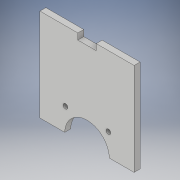
# Autodesk Inventor part: side_plate_top
Saved by Autodesk Inventor 2017 (Build 210142000, 142)
## iProperties
Created: 2017-07-18
Part Number: side_plate_top
Material: Generic
Document SubType Name: Modeling
Designer: millerid
Density: 1 g/cm^3
Appearance: Default
Author: millerid
Autodesk Inventor part; units mm, degrees
ref_plane "YZ Plane" through (0, 0, 0) normal (1, 0, 0) x (0, 1, 0)
ref_plane "XZ Plane" through (0, 0, 0) normal (0, 1, 0) x (-1, 0, 0)
ref_plane "XY Plane" through (0, 0, 0) normal (0, 0, 1) x (1, 0, 0)
sketch "Sketch1" plane through (0, 0, 0) normal (0, 0, 1) x (1, 0, 0)
  line L0 (20.2032, 59.7234) -> (20.2032, 63)
  line L1 (20.2032, 63) -> (0, 63)
  line L2 (0, 63) -> (0, 60)
  line L3 (30, 59.7234) -> (30, 63)
  line L4 (30, 63) -> (50.2032, 63)
  line L5 (50.2032, 63) -> (50.2032, 60)
  line L6 (30, 59.7234) -> (20.2032, 59.7234)
  circle A0 centre (13.6016, 25.8766) radius 1.25
  circle A1 centre (36.5, 25.6) radius 1.25
  line L7 (20.2032, 59.7234) -> (20.2032, 63)
  line L8 (20.2032, 63) -> (0, 63)
  line L9 (0, 63) -> (0, 60)
  line L10 (30, 59.7234) -> (30, 63)
  line L11 (30, 63) -> (50.2032, 63)
  line L12 (50.2032, 63) -> (50.2032, 60)
  line L13 (30, 59.7234) -> (20.2032, 59.7234)
  circle A2 centre (13.6016, 25.8766) radius 1.25
  circle A3 centre (36.5, 25.6) radius 1.25
  line L14 (0, 60) -> (0, 13.648)
  line L15 (50.2032, 60) -> (50.2032, 13.648)
  line L16 (0, 13.648) -> (13.2196, 13.648)
  line L17 (50.2032, 13.648) -> (36.9836, 13.648)
  arc A4 (36.9836, 13.648) -> (13.2196, 13.648) centre (25.1016, 13.3298) ccw
  point P0 (0, 0)
  dimension "d0" = 20.2032
  dimension "d1" = 3.2766
  dimension "d2" = 20.2032
  dimension "d3" = 2.5
  dimension "d4" = 2.5
  dimension "d7" = 20.2032
  dimension "d8" = 3.2766
  dimension "d9" = 20.2032
  dimension "d10" = 2.5
  dimension "d11" = 2.5
  dimension "d14" = 46.352
  dimension "d15" = 13.2196
  dimension "d16" = 13.2196
  constraints: 36 end point, 5 centre point, 4 horizontal, 4 parallel, 2 point on circle, 2 point on line, 2 vertical
  measures "d0" distance of L2.start L0.end
  measures "d1" distance of L0.end L6.end
  measures "d2" distance of L3.end L5.start
  measures "d3" diameter of A0
  measures "d4" diameter of A1
  measures "d7" distance of L9.start L7.end
  measures "d8" distance of L7.end L13.end
  measures "d9" distance of L10.end L12.start
  measures "d10" diameter of A2
  measures "d11" diameter of A3
  measures "d14" distance of L9.end L14.end
  measures "d15" distance of L14.end L16.end
  measures "d16" distance of L15.end L17.end
extrude "Extrusion1" add sketch "Sketch1" along normal blind 3.175
equation "\"d0\" = d5"
equation "\"d1\" = d6"
equation "\"d2\" = d5"
equation "\"d7\" = d12"
equation "\"d8\" = d13"
equation "\"d9\" = d12"
equation "\"d16\" = d15"
equation "\"d5\" = 20.2032"
equation "\"d6\" = 3.2766"
equation "\"d12\" = 20.2032"
equation "\"d13\" = 3.2766"
body "Solid1"
